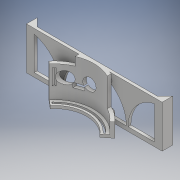
# Autodesk Inventor part: Mount US&.IRipt
Saved by Autodesk Inventor 2018.1 (Build 221171000, 171)
## iProperties
Created: 2019-01-27
Part Number: Mount US&.IRipt
Material: Типовые
Document SubType Name: Modeling
Designer: kostya
Density: 1 g/cm^3
Appearance: По умолчанию
Author: kostya
Autodesk Inventor part; units mm, degrees
ref_plane "YZ Plane" through (0, 0, 0) normal (1, 0, 0) x (0, 1, 0)
ref_plane "XZ Plane" through (0, 0, 0) normal (0, 1, 0) x (-1, 0, 0)
ref_plane "XY Plane" through (0, 0, 0) normal (0, 0, 1) x (1, 0, 0)
sketch "Эскиз1" plane through (0, 0, 0) normal (0, 0, 1) x (1, 0, 0)
  circle A0 centre (0, 0) radius 2.95 construction
  arc A1 (46.5372, 39.0493) -> (-46.5372, 39.0493) centre (0, 0) ccw
  arc A2 (42.7836, 35.8997) -> (-42.7836, 35.8997) centre (0, 0) ccw
  line L0 (0, 0) -> (-46.5372, 39.0493) construction
  line L1 (0, 0) -> (-60.75, 0) construction
  line L2 (0, 0) -> (46.5372, 39.0493) construction
  line L3 (0, 0) -> (60.75, 0) construction
  line L4 (-46.5372, 39.0493) -> (-42.7836, 35.8997)
  line L5 (46.5372, 39.0493) -> (42.7836, 35.8997)
  dimension "d0" = 5.9
  dimension "d2" = 4.9
  dimension "d8" = 40
  dimension "d9" = 40
  constraints: 12 end point, 4 coincident, 4 point on circle, 3 centre point, 2 collinear, 2 point on line
  measures "d0" diameter of A0
  measures "d2" radial gap between concentric circles of A1 A2
  measures "d8" angle of L0 L1
  measures "d9" angle of L3 L2
extrude "Выдавливание1" add sketch "Эскиз1" along normal blind 60
sketch "Эскиз2" plane through (0, 0, 0) normal (0, 0, -1) x (-1, 0, 0)
  arc A0 (42.7836, 35.8997) -> (-42.7836, 35.8997) centre (0, 0) ccw projected
  arc A1 (35.1997, 29.5361) -> (-30.4612, 34.4023) centre (0, 0) ccw
  line L0 (55.85, 0) -> (60.75, 0) projected
  line L1 (42.7836, 35.8997) -> (35.1997, 29.5361)
  line L2 (46.5372, 39.0493) -> (59.3372, 39.0493) construction
  line L3 (-42.7836, 35.8997) -> (-36.7318, 30.8217)
  arc A2 (-30.4612, 34.4023) -> (-35.1997, 29.5361) centre (0, 0) ccw
  arc A3 (42.7836, 35.8997) -> (-42.7836, 35.8997) centre (0, 0) ccw
  arc A4 (35.1997, 29.5361) -> (-35.1997, 29.5361) centre (0, 0) ccw
  line L4 (-35.1997, 29.5361) -> (-42.7746, 35.8922)
  line L5 (42.7836, 35.8997) -> (35.1997, 29.5361)
  arc A5 (42.7836, 35.8997) -> (-42.7836, 35.8997) centre (0, 0) ccw
  arc A6 (35.1997, 29.5361) -> (-35.1997, 29.5361) centre (0, 0) ccw
  line L6 (42.7836, 35.8997) -> (35.1997, 29.5361)
  line L7 (-42.7836, 35.8997) -> (-35.1997, 29.5361)
  dimension "d5" = 9.9
  dimension "d10" = 140
  constraints: 14 end point, 13 point on circle, 6 centre point, 5 coincident, 3 collinear, 1 horizontal, 1 point on line
  measures "d5" radial gap between concentric circles of A0 A1
  measures "d10" angle of L1 L2
extrude "Выдавливание3" add sketch "Эскиз2" against normal blind 4
ref_plane "РабПлоскость1" through (-42.7836, 35.8997, 0) normal (0, 1, 0) x (0, 0, 1)
sketch "Эскиз3" plane through (-42.7836, 35.8997, 0) normal (0, 1, 0) x (0, 0, 1)
  line L0 (32, 0) -> (32, 85.5672) construction
  line L1 (60, 42.7836) -> (4, 42.7836) construction
  line L2 (32, 3.6543) -> (32, 46.3606) construction
  line L3 (32, 85.5672) -> (32, 42.7836) construction
  line L4 (32, 25.0075) -> (32, 46.3606) construction
  line L5 (43.05, 1.8575) -> (20.95, 1.8575)
  line L6 (20.95, 48.1575) -> (43.05, 48.1575)
  line L7 (43.05, 48.1575) -> (43.05, 1.8575)
  line L8 (43.05, 1.8575) -> (20.95, 48.1575) construction
  line L9 (20.95, 1.8575) -> (43.05, 48.1575) construction
  line L10 (32, 48.1575) -> (32, 46.2575) construction
  line L11 (32, 46.2575) -> (32, 29.7961) construction
  line L12 (20.95, 38.0461) -> (23.25, 38.0461) construction
  line L13 (43.05, 38.0461) -> (40.45, 38.0461) construction
  line L14 (40.45, 38.0461) -> (40.45, 40.0461) construction
  line L15 (32, 46.2575) -> (34, 46.2575) construction
  line L16 (23.25, 38.0461) -> (23.25, 40.0461) construction
  arc A0 (27.4209, 30.2857) -> (26.0786, 31.2816) centre (31.85, 37.6575) ccw
  line L17 (32, 25.0075) -> (43.05, 25.0075) construction
  arc A1 (26.0786, 18.7333) -> (27.4209, 19.7293) centre (31.85, 12.3575) ccw
  line L18 (43.05, 25.0075) -> (26.8207, 25.0075) construction
  line L19 (23.25, 1.8575) -> (23.25, 19.8575) construction
  line L20 (23.25, 48.1575) -> (23.25, 30.1575) construction
  line L21 (20.95, 18.7333) -> (26.0786, 18.7333)
  line L22 (27.4209, 19.7293) -> (27.4209, 30.2857)
  line L23 (26.0786, 31.2816) -> (20.95, 31.2816)
  line L24 (20.95, 1.8575) -> (20.95, 18.7333)
  line L25 (20.95, 31.2816) -> (20.95, 48.1575)
  line L26 (20.95, 1.8575) -> (43.05, 1.8575)
  line L27 (43.05, 1.8575) -> (43.05, 48.1575)
  line L28 (43.05, 48.1575) -> (20.95, 48.1575)
  line L29 (20.95, 1.8575) -> (43.05, 48.1575) construction
  line L30 (43.05, 1.8575) -> (20.95, 48.1575) construction
  line L31 (20.95, 48.1575) -> (20.95, 31.2816)
  line L32 (20.95, 18.7333) -> (20.95, 1.8575)
  arc A2 (26.0786, 18.7333) -> (27.4209, 19.7293) centre (31.85, 12.3575) ccw
  arc A3 (27.4209, 30.2857) -> (26.0786, 31.2816) centre (31.85, 37.6575) ccw
  line L33 (26.0786, 18.7333) -> (20.95, 18.7333)
  line L34 (20.95, 18.7333) -> (20.95, 31.2816)
  point P0 (0, 42.7836)
  dimension "d13" = 22.1
  dimension "d14" = 46.3
  dimension "d15" = 1.9
  dimension "d17" = 2.3
  dimension "d18" = 2.6
  dimension "d19" = 2
  dimension "d20" = 2
  dimension "d21" = 2
  dimension "d22" = 18
  dimension "d23" = 18
  constraints: 70 end point, 11 parallel, 8 point on circle, 7 midpoint, 6 point on line, 4 centre point, 4 horizontal, 4 perpendicular, 3 tangent, 3 vertical, 2 coincident, 2 collinear, 2 concentric, 1 symmetric about line, 1 other
  measures "d13" distance of L6.start L6.end
  measures "d14" distance of L5.end L6.start
  measures "d15" distance of L10.start L10.end
  measures "d17" distance of L12.start L12.end
  measures "d18" distance of L13.start L13.end
  measures "d19" distance of L13.end L14.end
  measures "d20" distance of L10.end L15.end
  measures "d21" distance of L12.end L16.end
  measures "d22" distance of L19.start L19.end
  measures "d23" distance of L20.start L20.end
extrude "Выдавливание4" cut sketch "Эскиз3" along normal up to next contours L34 L23 A0 L22 A1 L21
extrude "Выдавливание5" cut sketch "Эскиз3" along normal mid plane 10 contours L5 L24 L21 A1 L22 A0 L23 L25 L6 L7
ref_plane "РабПлоскость2" through (0, 60.75, 0) normal (0, 1, 0) x (-1, 0, 0)
sketch "Эскиз4" plane through (0, 60.75, 0) normal (0, 1, 0) x (-1, 0, 0)
  line L0 (24.0503, 20.95) -> (11.502, 20.95) projected
  line L1 (11.502, 20.95) -> (11.502, 26.0786) projected
  line L2 (12.4979, 27.4209) -> (23.0543, 27.4209) projected
  line L3 (24.0503, 26.0786) -> (24.0503, 20.95) projected
  line L4 (46.5372, 0) -> (-46.5372, 0) projected
  line L5 (46.5372, 0) -> (46.5372, 60) projected
  line L6 (-46.5372, 60) -> (-46.5372, 60) projected
  line L7 (-46.5372, 0) -> (-46.5372, 60) projected
  line L8 (-42.7836, 60) -> (42.7836, 60) construction
  line L9 (-46.5372, 60) -> (-46.5372, 60) construction
  line L10 (-46.5372, 0) -> (46.5372, 0) construction
  line L11 (-41.7686, 26.25) -> (-1.0186, 26.25) construction
  line L12 (-1.0186, 33.75) -> (-41.7686, 33.75) construction
  line L13 (-39.2464, 27.225) -> (-3.422, 32.7935) construction
  line L14 (-1.9618, 26.9795) -> (-39.2464, 32.775) construction
  line L15 (-45.5186, 30) -> (-38.0186, 30) construction
  circle A0 centre (-41.7686, 30) radius 3.75 construction
  line L16 (-38.0186, 30) -> (-3.2725, 30) construction
  circle A1 centre (-41.7686, 30) radius 1.5 construction
  line L17 (-21.3936, 33.75) -> (-21.3936, 26.25) construction
  circle A2 centre (-1.0186, 30) radius 3.75 construction
  circle A3 centre (-1.0186, 30) radius 1.5 construction
  circle A4 centre (-41.7686, 30) radius 3.75 construction
  circle A5 centre (-41.7686, 30) radius 1.5 construction
  circle A6 centre (-1.0186, 30) radius 3.75 construction
  circle A7 centre (-1.0186, 30) radius 1.5 construction
  line L18 (-21.3936, 33.75) -> (-21.3936, 26.25) construction
  circle A8 centre (-21.3936, 9.625) radius 3.75
  circle A9 centre (-21.3936, 9.625) radius 3.75
  line L19 (-21.3936, 5.875) -> (-21.3936, 13.375) construction
  line L20 (-25.1436, 30) -> (-17.6436, 30) construction
  line L21 (-25.1436, 30) -> (-17.6436, 30) construction
  line L22 (-21.3936, 13.375) -> (-21.3936, 48.1211) construction
  line L23 (-18.6186, 12.1472) -> (-24.1871, 47.9716) construction
  line L24 (-18.3731, 49.4318) -> (-24.1686, 12.1472) construction
  line L25 (-17.6436, 9.625) -> (-17.6436, 50.375) construction
  line L26 (-25.1436, 50.375) -> (-25.1436, 9.625) construction
  circle A10 centre (-21.3936, 50.375) radius 1.5
  circle A11 centre (-21.3936, 50.375) radius 3.75
  circle A12 centre (-21.3936, 50.375) radius 3.75
  circle A13 centre (-21.3936, 50.375) radius 1.5
  circle A14 centre (-21.3936, 9.625) radius 1.5
  circle A15 centre (-21.3936, 9.625) radius 1.5
  point P0 (0, 0)
  point P1 (-21.3936, 30)
  point P2 (-21.3936, 30)
  dimension "d31" = 7.5
  dimension "d32" = 3
  dimension "d36" = 90
  constraints: 32 end point, 13 coincident, 12 centre point, 12 point on circle, 4 point on line, 3 midpoint, 2 parallel, 2 symmetric about line, 1 concentric, 1 horizontal, 1 horizontal alignment, 1 perpendicular, 1 vertical alignment, 55 other
  measures "d31" distance of L15.start L15.end
  measures "d32" diameter of A1
extrude "Выдавливание6" add sketch "Эскиз4" against normal up to next
sketch "Эскиз5" plane through (0, 0, 4) normal (0, 0, 1) x (1, 0, 0)
  arc A0 (42.7836, 35.8997) -> (-42.7836, 35.8997) centre (0, 0) ccw projected
  line L0 (-42.7836, 35.8997) -> (-35.1997, 29.5361) projected
  arc A1 (35.1997, 29.5361) -> (-35.1997, 29.5361) centre (0, 0) ccw projected
  line L1 (35.1997, 29.5361) -> (42.7836, 35.8997) projected
  line L2 (-42.7836, 35.8997) -> (-35.1997, 29.5361) construction
  line L3 (-42.7836, 35.8997) -> (-39.7194, 33.3285) construction
  line L4 (-35.1997, 29.5361) -> (-37.4979, 31.4645) construction
  line L5 (35.1997, 29.5361) -> (42.7836, 35.8997) projected
  arc A2 (35.7998, 33.3838) -> (-35.7998, 33.3838) centre (0, 0) ccw
  arc A3 (37.9207, 35.3616) -> (-37.9207, 35.3616) centre (0, 0) ccw
  line L6 (-39.7194, 33.3285) -> (-37.4979, 31.4645)
  line L7 (0, 0) -> (-35.7998, 33.3838) construction
  line L8 (0, 0) -> (-37.4979, 31.4645) construction
  arc A4 (-37.9207, 35.3616) -> (-35.7998, 33.3838) centre (-36.3853, 34.882) ccw
  arc A5 (35.1997, 29.5361) -> (-35.1997, 29.5361) centre (0, 0) ccw construction
  line L9 (0, 45.95) -> (0, 0) construction
  arc A6 (35.7998, 33.3838) -> (37.9207, 35.3616) centre (36.3853, 34.882) ccw
  point P0 (37.4979, 31.4645)
  point P1 (39.7194, 33.3285)
  dimension "d40" = 4
  dimension "d41" = 3
  dimension "d42" = 3
  constraints: 12 end point, 10 point on circle, 6 point on line, 4 centre point, 3 coincident, 3 symmetric about line, 1 vertical, 1 other
  measures "d40" distance of L0.start L3.end
  measures "d41" distance of L0.end L4.end
  measures "d42" angle of L7 L8
extrude "Выдавливание7" cut sketch "Эскиз5" against normal blind 10 contours A2 A4 A3 A6
sketch "Эскиз6" plane through (0, 60.75, 0) normal (0, 1, 0) x (-1, 0, 0)
  line L0 (-46.5372, 0) -> (46.5372, 0) projected
  line L1 (46.5372, 60) -> (-46.5372, 60) projected
  line L2 (-46.5372, 0) -> (-46.5372, 60) projected
  line L3 (46.5372, 0) -> (46.5372, 60) projected
  circle A0 centre (-21.3936, 9.625) radius 3.75 projected
  circle A1 centre (-21.3936, 50.375) radius 3.75 projected
  line L4 (35.1997, 0) -> (-35.1997, 0) projected
  line L5 (0, 60) -> (0, 0) construction
  line L6 (25.1436, 9.625) -> (25.1436, 5.875)
  line L7 (17.6436, 9.625) -> (25.1436, 9.625)
  line L8 (0, 5.875) -> (0, 0) construction
  line L9 (96, 0) -> (-96, 0)
  line L10 (-96, 0) -> (-96, 5.875)
  line L11 (96, 5.875) -> (96, 0)
  line L12 (96, 0) -> (-96, 5.875) construction
  line L13 (-96, 0) -> (96, 5.875) construction
  line L14 (-96, 5.875) -> (-25.1436, 5.875)
  arc A2 (-25.1436, 9.625) -> (-17.6436, 9.625) centre (-21.3936, 9.625) ccw
  line L15 (-17.6436, 5.875) -> (17.6436, 5.875)
  line L16 (25.1436, 5.875) -> (96, 5.875)
  line L17 (-25.1436, 9.625) -> (-25.1436, 5.875)
  line L18 (-17.6436, 9.625) -> (-17.6436, 5.875)
  line L19 (17.6436, 9.625) -> (17.6436, 5.875)
  line L20 (-46.5372, 30) -> (46.5372, 30) construction
  line L21 (-46.5372, 60) -> (46.5372, 60)
  circle A3 centre (-21.3936, 50.375) radius 3.75
  line L22 (35.1997, 60) -> (-35.1997, 60)
  line L23 (25.1436, 50.375) -> (25.1436, 54.125)
  line L24 (17.6436, 50.375) -> (25.1436, 50.375)
  line L25 (0, 54.125) -> (0, 60) construction
  line L26 (96, 60) -> (-96, 60)
  line L27 (-96, 60) -> (-96, 54.125)
  line L28 (96, 54.125) -> (96, 60)
  line L29 (96, 60) -> (-96, 54.125) construction
  line L30 (-96, 60) -> (96, 54.125) construction
  line L31 (-96, 54.125) -> (-25.1436, 54.125)
  arc A4 (-17.6436, 50.375) -> (-25.1436, 50.375) centre (-21.3936, 50.375) ccw
  line L32 (-17.6436, 54.125) -> (17.6436, 54.125)
  line L33 (25.1436, 54.125) -> (96, 54.125)
  line L34 (-25.1436, 50.375) -> (-25.1436, 54.125)
  line L35 (-17.6436, 50.375) -> (-17.6436, 54.125)
  line L36 (17.6436, 50.375) -> (17.6436, 54.125)
  point P0 (-17.6436, 0)
  point P1 (0, 2.9375)
  point P2 (-17.6436, 60)
  point P3 (0, 57.0625)
  dimension "d45" = 192
  constraints: 64 end point, 21 symmetric about line, 8 midpoint, 8 point on circle, 5 parallel, 3 centre point, 3 point on line, 2 coincident, 2 horizontal, 2 perpendicular, 1 collinear, 1 concentric, 1 tangent, 1 vertical, 2 other
  measures "d45" distance of L10.end L11.start
extrude "Выдавливание8" add sketch "Эскиз6" against normal blind 4 contours L2 L14 L17 A0 L18 L15 L19 L7 L6 L16 L3 L0 | L9 L10 L14 L2 | L31 L27 L26 L2 | L2 L1 L3 L33 L23 L24 L36 L32 L35 A1 L34 L31 | L3 L16 L11 L9 | L3 L26 L28 L33
sketch "Эскиз9" plane through (0, 60.75, 0) normal (0, 1, 0) x (1, 0, 0)
  circle A0 centre (21.3936, -50.375) radius 1.5 projected
  arc A1 (25.1436, -50.375) -> (17.6436, -50.375) centre (21.3936, -50.375) ccw projected
  line L0 (17.6436, -50.375) -> (17.6436, -54.125) projected
  line L1 (17.6436, -54.125) -> (0, -54.125) projected
  line L2 (0, -54.125) -> (-17.6436, -54.125) projected
  line L3 (-17.6436, -54.125) -> (-17.6436, -50.375) projected
  line L4 (-17.6436, -50.375) -> (-25.1436, -50.375) projected
  line L5 (-25.1436, -50.375) -> (-25.1436, -54.125) projected
  line L6 (-25.1436, -54.125) -> (-96, -54.125) projected
  line L7 (-96, -54.125) -> (-96, -60) projected
  line L8 (-96, -60) -> (96, -60) projected
  line L9 (96, -60) -> (96, -54.125) projected
  line L10 (96, -54.125) -> (25.1436, -54.125) projected
  line L11 (25.1436, -54.125) -> (25.1436, -50.375) projected
  circle A2 centre (21.3936, -9.625) radius 1.5 projected
  arc A3 (17.6436, -9.625) -> (25.1436, -9.625) centre (21.3936, -9.625) ccw projected
  line L12 (25.1436, -9.625) -> (25.1436, -5.875) projected
  line L13 (25.1436, -5.875) -> (96, -5.875) projected
  line L14 (96, -5.875) -> (96, 0) projected
  line L15 (96, 0) -> (-96, 0) projected
  line L16 (-96, 0) -> (-96, -5.875) projected
  line L17 (-96, -5.875) -> (-25.1436, -5.875) projected
  line L18 (-25.1436, -5.875) -> (-25.1436, -9.625) projected
  line L19 (-25.1436, -9.625) -> (-17.6436, -9.625) projected
  line L20 (-17.6436, -9.625) -> (-17.6436, -5.875) projected
  line L21 (-17.6436, -5.875) -> (0, -5.875) projected
  line L22 (0, -5.875) -> (17.6436, -5.875) projected
  line L23 (17.6436, -5.875) -> (17.6436, -9.625) projected
  line L24 (96, -5.875) -> (96, 0) projected
  arc A4 (47.75, -5.875) -> (96, -54.125) centre (96, -5.875) ccw
  line L25 (46.5372, 0) -> (46.5372, -60) construction
  line L26 (46.5372, -54.125) -> (46.5372, -5.875) construction
  arc A5 (17.6436, -49.521) -> (17.7548, -49.4684) centre (-2.9256, -5.875) ccw
  arc A6 (22.5956, -46.8229) -> (45.3244, -5.875) centre (-2.9256, -5.875) ccw
  line L27 (47.75, -5.875) -> (45.3244, -5.875) construction
  line L28 (25.1436, -5.875) -> (96, -5.875) construction
  line L29 (96, -54.125) -> (25.1436, -54.125) construction
  line L30 (47.75, -5.875) -> (45.3244, -5.875)
  line L31 (96, -5.875) -> (25.1436, -5.875) projected
  line L32 (96, -54.125) -> (25.1436, -54.125) projected
  line L33 (96, -54.125) -> (25.1436, -54.125)
  line L34 (25.1436, -54.125) -> (25.1436, -50.375)
  arc A7 (25.1436, -50.375) -> (17.6436, -50.375) centre (21.3936, -50.375) ccw projected
  arc A8 (25.1436, -50.375) -> (22.5956, -46.8229) centre (21.3936, -50.375) ccw
  line L35 (42.7836, -60) -> (-42.7836, -60) construction
  line L36 (0, -60) -> (0, 0) construction
  line L37 (-96, -54.125) -> (-25.1436, -54.125)
  arc A9 (-96, -54.125) -> (-47.75, -5.875) centre (-96, -5.875) ccw
  line L38 (-46.5372, 0) -> (-46.5372, -60) construction
  line L39 (-46.5372, -60) -> (-46.5372, 0) construction
  arc A10 (-45.3244, -5.875) -> (2.9256, -54.125) centre (2.9256, -5.875) ccw
  line L40 (2.9256, -54.125) -> (-17.6436, -54.125)
  line L41 (17.6436, -54.125) -> (0, -54.125) projected
  line L42 (-17.6436, -54.125) -> (-25.1436, -54.125)
  line L43 (-45.3244, -5.875) -> (-47.75, -5.875)
  point P0 (-2.9256, -54.125)
  constraints: 24 end point, 15 point on circle, 8 symmetric about line, 6 centre point, 6 collinear, 5 point on line, 2 tangent, 2 vertical, 1 coincident, 1 horizontal, 1 midpoint, 1 perpendicular, 2 other
extrude "Выдавливание12" add sketch "Эскиз9" against normal up to surface (4 mm away) contours A1 A6 L13 A4 L10 L11 | L1 L2 L3 L4 L5 L6 A9 L17 A10
extrude "Выдавливание13" cut sketch "Эскиз3" along normal up to surface (24.8503 mm away) contours L34 L23 A0 L22 A1 L21
sketch "Эскиз10" plane through (-96, 56.75, 5.875) normal (0, 0, 1) x (1, 0, 0)
  line L0 (0, 0) -> (15, 0)
  line L1 (48.25, 0) -> (0, 0) projected
  line L2 (15, 0) -> (0, 15)
  line L3 (0, 15) -> (0, 0)
  point P0 (96, -56.75)
  dimension "d60" = 15
  dimension "d61" = 45
  constraints: 6 end point, 1 perpendicular, 1 point on line
  measures "d60" distance of L0.start L0.end
  measures "d61" angle of L2 L0
extrude "Выдавливание14" add sketch "Эскиз10" against normal up to surface (5.875 mm away)
ref_plane "РабПлоскость4" through (0, 56.75, 60) normal (-1, 0, 0) x (0, 0, 1)
ref_plane "РабПлоскость5" through (0, 0, 30) normal (0, 0, -1) x (-1, 0, 0)
mirror "Зеркальное отражение3" about plane through (0, 0, 30) normal (0, 0, -1) of "Выдавливание14"
mirror "Зеркальное отражение4" about plane through (0, 56.75, 60) normal (-1, 0, 0) of "Выдавливание14", "Зеркальное отражение3"
sketch "Эскиз11" plane through (-96, 56.75, 5.875) normal (0, 0, 1) x (1, 0, 0)
  line L0 (48.25, 0) -> (0, 0) projected
  line L1 (48.25, 0) -> (48.25, 4) projected
  line L2 (11, 4) -> (48.25, 4) projected
  line L3 (11, 4) -> (0, 15) projected
  line L4 (0, 15) -> (0, 0) projected
  line L5 (11, 4) -> (0, 15) projected
  line L6 (11, 4) -> (11, 0)
  line L7 (48.25, 0) -> (0, 0) projected
  line L8 (181, 4) -> (11, 4) projected
  line L9 (11, 4) -> (0, 15)
  line L10 (0, 15) -> (0, 0) projected
  line L11 (0, 15) -> (0, 0)
  line L12 (0, 0) -> (11, 0)
  line L13 (11, 4) -> (11, 0)
  line L14 (0, 0) -> (0, 15)
  line L15 (11, 4) -> (0, 15)
  line L16 (11, 0) -> (0, 0)
  point P0 (96, -56.75)
  constraints: 16 end point, 4 perpendicular, 2 collinear, 1 point on line
extrude "Выдавливание15" add sketch "Эскиз11" along normal up to next contours L0 L4 L3 L6
mirror "Зеркальное отражение5" about plane through (0, 56.75, 60) normal (-1, 0, 0) of "Выдавливание15"
sketch "Эскиз12" plane through (0, 0, 60) normal (0, 0, 1) x (1, 0, 0)
  line L0 (0, -14.35) -> (0, 86.1) projected
  line L1 (-11.502, 54.6528) -> (5.698, 54.6528) construction
  line L2 (-96, 71.75) -> (-85, 60.75) projected
  line L3 (-96, 56.75) -> (-96, 71.75) projected
  line L4 (-21.6795, 56.75) -> (-96, 56.75) projected
  arc A0 (-21.6795, 56.75) -> (-46.5372, 39.0493) centre (0, 0) ccw projected
  line L5 (-46.5372, 39.0493) -> (-42.7836, 35.8997) projected
  arc A1 (42.7836, 35.8997) -> (-42.7836, 35.8997) centre (0, 0) ccw projected
  line L6 (42.7836, 35.8997) -> (46.5372, 39.0493) projected
  arc A2 (46.5372, 39.0493) -> (21.6795, 56.75) centre (0, 0) ccw projected
  line L7 (96, 56.75) -> (21.6795, 56.75) projected
  line L8 (96, 56.75) -> (96, 71.75) projected
  line L9 (96, 71.75) -> (85, 60.75) projected
  line L10 (-85, 60.75) -> (85, 60.75) projected
  arc A3 (17.6436, 58.1315) -> (2.9256, 60.6795) centre (0, 0) ccw projected
  line L11 (-21.6795, 56.75) -> (-21.6795, 51.4706)
  line L12 (-21.6795, 56.75) -> (-16.4001, 56.75) construction
  arc A4 (46.5372, 39.0493) -> (21.6795, 56.75) centre (0, 0) ccw projected
  arc A5 (21.6795, 56.75) -> (21.6795, 56.75) centre (0, 0) ccw
  arc A6 (42.7836, 35.8997) -> (-42.7836, 35.8997) centre (0, 0) ccw projected
  arc A7 (42.7836, 35.8997) -> (25.1436, 49.87) centre (0, 0) ccw
  arc A8 (-21.6795, 56.75) -> (-46.5372, 39.0493) centre (0, 0) ccw
  arc A9 (-21.6795, 51.4706) -> (-42.7836, 35.8997) centre (0, 0) ccw
  arc A10 (-21.6795, 56.75) -> (-46.5372, 39.0493) centre (0, 0) ccw projected
  line L13 (-46.5372, 39.0493) -> (-42.7836, 35.8997) projected
  line L14 (-46.5372, 39.0493) -> (-42.7836, 35.8997)
  line L15 (46.5372, 39.0493) -> (42.7836, 35.8997)
  arc A11 (46.5372, 39.0493) -> (25.1436, 55.3025) centre (0, 0) ccw
  line L16 (42.7836, 35.8997) -> (46.5372, 39.0493)
  arc A12 (46.5372, 39.0493) -> (25.1436, 55.3025) centre (0, 0) ccw
  arc A13 (42.7836, 35.8997) -> (25.1436, 49.87) centre (0, 0) ccw
  line L17 (21.6795, 56.75) -> (25.1436, 56.75) projected
  line L18 (25.1436, 55.3025) -> (25.1436, 49.87)
  arc A14 (42.7836, 35.8997) -> (-42.7836, 35.8997) centre (0, 0) ccw projected
  point P0 (22.5956, 56.75)
  dimension "d68" = 90
  constraints: 14 end point, 14 point on circle, 6 centre point, 5 concentric, 2 collinear, 2 horizontal, 2 point on line, 1 perpendicular, 1 vertical, 4 other
  measures "d68" angle of L11 L12
extrude "Выдавливание17" cut sketch "Эскиз12" against normal blind 40 contours L18 A2 L6 A1
extrude "Выдавливание18" cut sketch "Эскиз12" against normal blind 12 contours A1 L5 A0 L11
